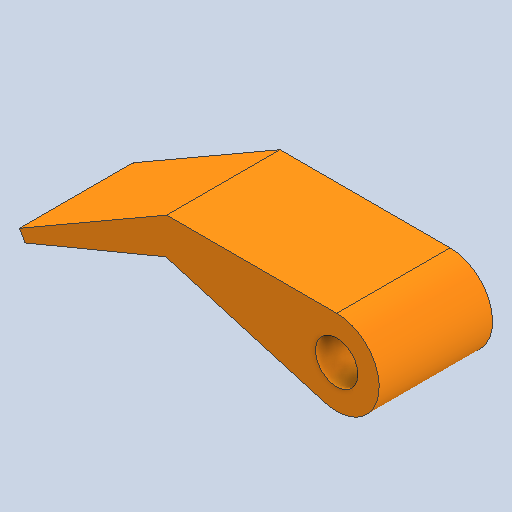
# Autodesk Inventor part: Claw
Saved by Autodesk Inventor 2024 (Build 280153000, 153)
## iProperties
Created: 2023-06-06
Part Number: Claw
Material: Steel, Alloy
Document SubType Name: Modeling
Designer: vilas
Density: 7.73 g/cm^3
Appearance: Semi-Polished
Author: vilas
Autodesk Inventor part; units mm, degrees
ref_plane "YZ Plane" through (0, 0, 0) normal (1, 0, 0) x (0, 1, 0)
ref_plane "XZ Plane" through (0, 0, 0) normal (0, 1, 0) x (-1, 0, 0)
ref_plane "XY Plane" through (0, 0, 0) normal (0, 0, 1) x (1, 0, 0)
sketch "Sketch1" plane through (0, 0, 0) normal (0, 0, 1) x (1, 0, 0)
  arc A0 (-2.1175, -7.1949) -> (0, 7.5) centre (0, 0) ccw
  circle A1 centre (0, 0) radius 3.75
  line L0 (0, 7.5) -> (-30, 7.5)
  line L1 (-30, 7.5) -> (-55.9808, -7.5)
  line L2 (-55.9808, -7.5) -> (-54.9808, -9.2321)
  line L3 (-54.9808, -9.2321) -> (-30.1469, 1.0545)
  line L4 (-30.1469, 1.0545) -> (-2.1175, -7.1949)
  dimension "d0" = 15
  dimension "d1" = 7.5
  dimension "d2" = 30
  dimension "d3" = 30
  dimension "d4" = 150
  dimension "d5" = 2
  dimension "d6" = 97.5
  dimension "d7" = 6.4455
  constraints: 10 end point, 2 centre point, 2 coincident, 2 point on circle, 2 tangent, 1 horizontal, 1 perpendicular
  measures "d0" diameter of A0
  measures "d1" diameter of A1
  measures "d2" distance of L0.start L0.end
  measures "d3" distance of L0.end L1.end
  measures "d4" angle of L1 L0
  measures "d5" distance of L1.end L2.end
  measures "d6" angle of L3 L2
  measures "d7" vertical distance of L3.end L0.end
extrude "Extrusion1" add sketch "Sketch1" along normal mid plane 20
body "Solid1"
